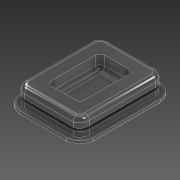
# Autodesk Inventor part: TAPAV2
Saved by Autodesk Inventor 2021 (Build 250183000, 183)
## iProperties
Created: 2022-08-14
Part Number: TAPAV2
Material: Plástico ABS
Document SubType Name: Modeling
Designer: PC
Density: 1.06 g/cm^3
Appearance: Gris oscuro
Author: PC
Autodesk Inventor part; units mm, degrees
ref_plane "YZ Plane" through (0, 0, 0) normal (1, 0, 0) x (0, 1, 0)
ref_plane "XZ Plane" through (0, 0, 0) normal (0, 1, 0) x (-1, 0, 0)
ref_plane "XY Plane" through (0, 0, 0) normal (0, 0, 1) x (1, 0, 0)
sketch "Boceto1" plane through (0, 0, 0) normal (0, 1, 0) x (-1, 0, 0)
  arc A0 (9.988, -9.8253) -> (15.988, -3.8253) centre (9.988, -3.8253) ccw
  line L0 (15.988, -3.8253) -> (15.988, 24.6747)
  arc A1 (15.988, 24.6747) -> (9.988, 30.6747) centre (9.988, 24.6747) ccw
  line L1 (9.988, 30.6747) -> (-9.862, 30.6747)
  arc A2 (-9.862, 30.6747) -> (-15.862, 24.6747) centre (-9.862, 24.6747) ccw
  line L2 (-15.862, 24.6747) -> (-15.862, -3.8253)
  arc A3 (-15.862, -3.8253) -> (-9.862, -9.8253) centre (-9.862, -3.8253) ccw
  line L3 (-9.862, -9.8253) -> (9.988, -9.8253)
  arc A4 (-13.862, -3.8253) -> (-9.862, -7.8253) centre (-9.862, -3.8253) ccw
  line L4 (-13.862, -3.8253) -> (-13.862, 24.6747)
  arc A5 (-10.9421, 28.6747) -> (-13.862, 24.6747) centre (-9.6623, 24.6747) ccw
  line L5 (-10.9421, 28.6747) -> (9.988, 28.6747)
  arc A6 (13.988, 24.6747) -> (9.988, 28.6747) centre (9.988, 24.6747) ccw
  line L6 (13.988, 24.6747) -> (13.988, -4.9054)
  arc A7 (9.988, -7.8253) -> (13.988, -4.9054) centre (9.988, -3.6255) ccw
  line L7 (9.988, -7.8253) -> (-9.862, -7.8253)
  line L8 (14.388, -4.9664) -> (14.388, 24.6747)
  arc A8 (14.388, 24.6747) -> (9.988, 29.0747) centre (9.988, 24.6747) ccw
  line L9 (9.988, 29.0747) -> (-11.0031, 29.0747)
  arc A9 (-11.0031, 29.0747) -> (-14.262, 24.6747) centre (-9.6623, 24.6747) ccw
  line L10 (-14.262, 24.6747) -> (-14.262, -3.8253)
  arc A10 (-14.262, -3.8253) -> (-9.862, -8.2253) centre (-9.862, -3.8253) ccw
  line L11 (-9.862, -8.2253) -> (9.988, -8.2253)
  arc A11 (9.988, -8.2253) -> (14.388, -4.9664) centre (9.988, -3.6255) ccw
  point P0 (0, 0)
  point P1 (0, 0)
  dimension "d0" = 27.85
  dimension "d1" = 40.5
  dimension "d2" = 6
  dimension "d3" = 2
  dimension "d4" = 2
  dimension "d5" = 2
  dimension "d6" = 2
  dimension "d7" = 2
  dimension "d8" = 0.4
  constraints: 24 end point, 24 point on circle, 12 centre point, 7 other
  measures "d0" distance between parallel lines of L4 L6
  measures "d1" distance between parallel lines of L3 L1
  measures "d2" radius of A0
  measures "d3" distance between parallel lines of L0 L6
  measures "d4" distance between parallel lines of L3 L7
  measures "d5" distance between parallel lines of L2 L4
  measures "d6" distance between parallel lines of L1 L5
  measures "d7" radial gap between concentric circles of A6 A1
  measures "d8" distance between parallel lines of L6 L8
extrude "Extrusión1" add sketch "Boceto1" along normal blind 4 contours L4 A5 L5 A6 L6 A7 L7 A4
extrude "Extrusión2" add sketch "Boceto1" along normal blind 2 contours L3 A3 L2 A2 L1 A1 L0 A0 | A11 L11 A10 L10 A9 L9 A8 L8
sketch "Boceto2" plane through (0, 4, 0) normal (0, 1, 0) x (1, 0, 0)
  line L0 (13.862, -24.6747) -> (13.862, 3.8253) projected
  arc A0 (13.862, 3.8253) -> (9.862, 7.8253) centre (9.862, 3.8253) ccw projected
  line L1 (9.862, 7.8253) -> (-9.988, 7.8253) projected
  arc A1 (-9.988, 7.8253) -> (-13.988, 4.9054) centre (-9.988, 3.6255) ccw projected
  line L2 (-13.988, 4.9054) -> (-13.988, -24.6747) projected
  arc A2 (-13.988, -24.6747) -> (-9.988, -28.6747) centre (-9.988, -24.6747) ccw projected
  line L3 (-9.988, -28.6747) -> (10.9421, -28.6747) projected
  arc A3 (10.9421, -28.6747) -> (13.862, -24.6747) centre (9.6623, -24.6747) ccw projected
  line L4 (-12.488, -24.6747) -> (-12.488, 4.6447)
  arc A4 (-9.988, 6.3253) -> (-12.488, 4.6447) centre (-9.988, 3.6255) ccw
  line L5 (-9.988, 6.3253) -> (9.862, 6.3253)
  arc A5 (12.362, 3.8253) -> (9.862, 6.3253) centre (9.862, 3.8253) ccw
  line L6 (12.362, 3.8253) -> (12.362, -24.6747)
  arc A6 (10.6815, -27.1747) -> (12.362, -24.6747) centre (9.6623, -24.6747) ccw
  line L7 (10.6815, -27.1747) -> (-9.988, -27.1747)
  arc A7 (-12.488, -24.6747) -> (-9.988, -27.1747) centre (-9.988, -24.6747) ccw
  point P0 (0, 0)
  dimension "d13" = 1.5
  constraints: 8 end point, 8 point on circle, 4 centre point, 7 other
  measures "d13" distance between parallel lines of L4 L2
extrude "Extrusión3" add sketch "Boceto2" along normal blind 1.3 contours L4 A4 L5 A5 L6 A6 L7 A7
sketch "Boceto3" plane through (0, 5.3, 0) normal (0, 1, 0) x (1, 0, 0)
  arc A0 (10.6815, -27.1747) -> (12.362, -24.6747) centre (9.6623, -24.6747) ccw projected
  line L0 (10.6815, -27.1747) -> (-9.988, -27.1747) projected
  arc A1 (-12.488, -24.6747) -> (-9.988, -27.1747) centre (-9.988, -24.6747) ccw projected
  line L1 (-12.488, -24.6747) -> (-12.488, 4.6447) projected
  arc A2 (-9.988, 6.3253) -> (-12.488, 4.6447) centre (-9.988, 3.6255) ccw projected
  line L2 (-9.988, 6.3253) -> (9.862, 6.3253) projected
  arc A3 (12.362, 3.8253) -> (9.862, 6.3253) centre (9.862, 3.8253) ccw projected
  line L3 (12.362, 3.8253) -> (12.362, -24.6747) projected
  line L4 (13.862, -24.6747) -> (13.862, 3.8253) projected
  arc A4 (13.862, 3.8253) -> (9.862, 7.8253) centre (9.862, 3.8253) ccw projected
  line L5 (9.862, 7.8253) -> (-9.988, 7.8253) projected
  arc A5 (-9.988, 7.8253) -> (-13.988, 4.9054) centre (-9.988, 3.6255) ccw projected
  line L6 (-13.988, 4.9054) -> (-13.988, -24.6747) projected
  arc A6 (-13.988, -24.6747) -> (-9.988, -28.6747) centre (-9.988, -24.6747) ccw projected
  line L7 (-9.988, -28.6747) -> (10.9421, -28.6747) projected
  arc A7 (10.9421, -28.6747) -> (13.862, -24.6747) centre (9.6623, -24.6747) ccw projected
  point P0 (0, 0)
extrude "Extrusión4" add sketch "Boceto3" along normal blind 4 contours L0 A1 L1 A2 L2 A3 L3 A0 | A7 L7 A6 L6 A5 L5 A4 L4
sketch "Boceto4" plane through (0, 9.3, 0) normal (0, 1, 0) x (1, 0, 0)
  arc A0 (13.862, 3.8253) -> (9.862, 7.8253) centre (9.862, 3.8253) ccw projected
  line L0 (9.862, 7.8253) -> (-9.988, 7.8253) projected
  arc A1 (-9.988, 7.8253) -> (-13.988, 4.9054) centre (-9.988, 3.6255) ccw projected
  line L1 (-13.988, 4.9054) -> (-13.988, -24.6747) projected
  arc A2 (-13.988, -24.6747) -> (-9.988, -28.6747) centre (-9.988, -24.6747) ccw projected
  line L2 (-9.988, -28.6747) -> (10.9421, -28.6747) projected
  arc A3 (10.9421, -28.6747) -> (13.862, -24.6747) centre (9.6623, -24.6747) ccw projected
  line L3 (13.862, -24.6747) -> (13.862, 3.8253) projected
  line L4 (-12.188, -24.6747) -> (-12.188, 4.5841)
  arc A4 (-9.988, 6.0253) -> (-12.188, 4.5841) centre (-9.988, 3.6255) ccw
  line L5 (-9.988, 6.0253) -> (9.862, 6.0253)
  arc A5 (12.062, 3.8253) -> (9.862, 6.0253) centre (9.862, 3.8253) ccw
  line L6 (12.062, 3.8253) -> (12.062, -24.6747)
  arc A6 (10.6209, -26.8747) -> (12.062, -24.6747) centre (9.6623, -24.6747) ccw
  line L7 (10.6209, -26.8747) -> (-9.988, -26.8747)
  arc A7 (-12.188, -24.6747) -> (-9.988, -26.8747) centre (-9.988, -24.6747) ccw
  line L8 (-7.2861, -0.8765) -> (-7.2861, -19.9729)
  line L9 (-5.2861, -21.9729) -> (5.1602, -21.9729)
  line L10 (7.1602, -19.9729) -> (7.1602, -0.8765)
  line L11 (5.1602, 1.1235) -> (-5.2861, 1.1235)
  arc A8 (-7.2861, -19.9729) -> (-5.2861, -21.9729) centre (-5.2861, -19.9729) ccw
  arc A9 (-5.2861, 1.1235) -> (-7.2861, -0.8765) centre (-5.2861, -0.8765) ccw
  arc A10 (7.1602, -0.8765) -> (5.1602, 1.1235) centre (5.1602, -0.8765) ccw
  arc A11 (5.1602, -21.9729) -> (7.1602, -19.9729) centre (5.1602, -19.9729) ccw
  point P0 (0, 0)
  dimension "d18" = 1.8
  dimension "d19" = 2
  constraints: 16 end point, 16 point on circle, 8 centre point, 8 tangent, 3 equal radius, 10 other
  measures "d18" distance between parallel lines of L4 L1
  measures "d19" radius of A8
extrude "Extrusión5" cut sketch "Boceto4" against normal blind 6 contours A9 L11 A10 L10 A11 L9 A8 L8
fillet "Empalme1" radius 2 8 edges at (-6.7003, 3.3, -0.5377) (-0.063, 3.3, -1.1235) (6.5744, 3.3, -0.5377) (7.1602, 3.3, 10.4247) (6.5744, 3.3, 21.3871) (-0.063, 3.3, 21.9729) (-6.7003, 3.3, 21.3871) (-7.2861, 3.3, 10.4247)
fillet "Empalme2" radius 2 8 edges at (-12.8164, 9.3, 27.5031) (-13.988, 9.3, 9.8847) (0.4771, 9.3, 28.6747) (-12.4641, 9.3, -7.0177) (12.6905, 9.3, -6.6537) (13.862, 9.3, 10.4247) (13.0544, 9.3, 27.1509) (-0.063, 9.3, -7.8253)
fillet "Empalme3" radius 1 8 edges at (-14.2306, 0, 28.9173) (-0.063, 0, 30.6747) (14.1047, 0, 28.9173) (15.862, 0, 10.4247) (14.1047, 0, -8.0679) (-0.063, 0, -9.8253) (-14.2306, 0, -8.0679) (-15.988, 0, 10.4247)
sketch "Boceto5" plane through (0, 0, 0) normal (0, -1, 0) x (1, 0, 0)
  line L0 (-2.8976, -4.217) -> (-2.8976, 9.8768) construction
  line L1 (-2.8976, 9.8768) -> (29.3615, 9.8768) construction
  line L2 (29.3615, 9.8768) -> (29.3615, -4.217) construction
  line L3 (29.3615, -4.217) -> (-2.8976, -4.217) construction
  line L4 (-2.8976, -3.5852) -> (-2.8976, -0.7989)
  spline S0 degree 2 poles (-2.8976, -0.7989) (-2.8976, -0.0973) (-2.7533, 0.7436) (-2.5941, 0.9923) knots 0 0 0 1 2 2 2
  spline S1 degree 2 poles (-2.5941, 0.9923) (-2.3304, 1.4053) (-1.4697, 1.8332) (-0.9124, 1.8332) knots 0 0 0 1 2 2 2
  spline S2 degree 2 poles (-0.9124, 1.8332) (-0.3651, 1.8332) (0.421, 1.4849) (0.6798, 1.1267) knots 0 0 0 1 2 2 2
  spline S3 degree 2 poles (0.6798, 1.1267) (0.8887, 0.8281) (1.0679, 0.052) (1.0679, -0.7491) knots 0 0 0 1 2 2 2
  line L5 (1.0679, -0.7491) -> (1.0679, -2.3015)
  line L6 (1.0679, -2.3015) -> (3.2024, -2.3015)
  line L7 (3.2024, -2.3015) -> (3.2024, -3.5852)
  line L8 (3.2024, -3.5852) -> (-2.8976, -3.5852)
  line L9 (-1.808, -0.8188) -> (-1.808, -2.3015)
  line L10 (-1.808, -2.3015) -> (-0.0118, -2.3015)
  line L11 (-0.0118, -2.3015) -> (-0.0118, -0.7392)
  spline S4 degree 2 poles (-0.0118, -0.7392) (-0.0118, -0.157) (-0.4547, 0.4052) (-0.9124, 0.4052) knots 0 0 0 1 2 2 2
  spline S5 degree 2 poles (-0.9124, 0.4052) (-1.4, 0.4052) (-1.808, -0.1471) (-1.808, -0.8188) knots 0 0 0 1 2 2 2
  line L12 (-2.8976, 3.9826) -> (0.7494, 3.9826)
  spline S6 degree 2 poles (0.7494, 3.9826) (1.6052, 3.9826) (2.2819, 4.5996) (2.2819, 5.3559) knots 0 0 0 1 2 2 2
  spline S7 degree 2 poles (2.2819, 5.3559) (2.2819, 6.1122) (1.6102, 6.7241) (0.7494, 6.7241) knots 0 0 0 1 2 2 2
  line L13 (0.7494, 6.7241) -> (-2.8976, 6.7241)
  line L14 (-2.8976, 6.7241) -> (-2.8976, 8.0078)
  line L15 (-2.8976, 8.0078) -> (0.7843, 8.0078)
  spline S8 degree 2 poles (0.7843, 8.0078) (1.4311, 8.0078) (2.2023, 7.8387) (2.4262, 7.6496) knots 0 0 0 1 2 2 2
  spline S9 degree 2 poles (2.4262, 7.6496) (2.8591, 7.2864) (3.267, 6.1768) (3.267, 5.3559) knots 0 0 0 1 2 2 2
  spline S10 degree 2 poles (3.267, 5.3559) (3.267, 4.5349) (2.8591, 3.4154) (2.4262, 3.0522) knots 0 0 0 1 2 2 2
  spline S11 degree 2 poles (2.4262, 3.0522) (2.2073, 2.8681) (1.4609, 2.7039) (0.7843, 2.7039) knots 0 0 0 1 2 2 2
  line L16 (0.7843, 2.7039) -> (-2.8976, 2.7039)
  line L17 (-2.8976, 2.7039) -> (-2.8976, 3.9826)
  spline S12 degree 2 poles (3.2024, 11.6698) (3.2024, 10.819) (2.9138, 9.9881) (2.5605, 9.6597) knots 0 0 0 1 2 2 2
  spline S13 degree 2 poles (2.5605, 9.6597) (2.2471, 9.3562) (1.451, 9.1074) (0.7295, 9.1074) knots 0 0 0 1 2 2 2
  line L18 (0.7295, 9.1074) -> (-2.8976, 9.1074)
  line L19 (-2.8976, 9.1074) -> (-2.8976, 10.3911)
  line L20 (-2.8976, 10.3911) -> (0.6847, 10.3911)
  spline S14 degree 2 poles (0.6847, 10.3911) (1.2221, 10.3911) (1.655, 10.4856) (1.7893, 10.6001) knots 0 0 0 1 2 2 2
  spline S15 degree 2 poles (1.7893, 10.6001) (2.0033, 10.7842) (2.1874, 11.3166) (2.1874, 11.7843) knots 0 0 0 1 2 2 2
  line L21 (2.1874, 11.7843) -> (2.1874, 13.2918)
  line L22 (2.1874, 13.2918) -> (3.2024, 13.2918)
  line L23 (3.2024, 13.2918) -> (3.2024, 11.6698)
  line L24 (-1.808, 19.1331) -> (-1.808, 15.9637)
  spline S16 degree 2 poles (-1.808, 15.9637) (-1.808, 15.4512) (-1.4249, 14.9736) (-1.0119, 14.9736) knots 0 0 0 1 2 2 2
  spline S17 degree 2 poles (-1.0119, 14.9736) (-0.6835, 14.9736) (-0.3502, 15.3816) (-0.3502, 15.7846) knots 0 0 0 1 2 2 2
  line L25 (-0.3502, 15.7846) -> (-0.3502, 17.4812)
  spline S18 degree 2 poles (-0.3502, 17.4812) (-0.3502, 18.5361) (0.4459, 19.4267) (1.3763, 19.4267) knots 0 0 0 1 2 2 2
  spline S19 degree 2 poles (1.3763, 19.4267) (2.3167, 19.4267) (3.2024, 18.3967) (3.2024, 17.2971) knots 0 0 0 1 2 2 2
  line L26 (3.2024, 17.2971) -> (3.2024, 13.879)
  line L27 (3.2024, 13.879) -> (2.1127, 13.879)
  line L28 (2.1127, 13.879) -> (2.1127, 17.0931)
  spline S20 degree 2 poles (2.1127, 17.0931) (2.1127, 17.6405) (1.7943, 18.0883) (1.4261, 18.0883) knots 0 0 0 1 2 2 2
  spline S21 degree 2 poles (1.4261, 18.0883) (1.043, 18.0883) (0.7196, 17.6753) (0.7196, 17.1777) knots 0 0 0 1 2 2 2
  line L29 (0.7196, 17.1777) -> (0.7196, 15.6652)
  spline S22 degree 2 poles (0.7196, 15.6652) (0.7196, 14.6104) (-0.1213, 13.6352) (-1.0318, 13.6352) knots 0 0 0 1 2 2 2
  spline S23 degree 2 poles (-1.0318, 13.6352) (-2.002, 13.6352) (-2.8976, 14.6601) (-2.8976, 15.7746) knots 0 0 0 1 2 2 2
  line L30 (-2.8976, 15.7746) -> (-2.8976, 19.1331)
  line L31 (-2.8976, 19.1331) -> (-1.808, 19.1331)
  spline S24 degree 2 poles (-1.8329, 22.9095) (-1.8329, 22.213) (-1.1363, 21.5015) (-0.4198, 21.4666) knots 0 0 0 1 2 2 2
  line L32 (-0.4198, 21.4666) -> (-0.4148, 25.0142)
  line L33 (-0.4148, 25.0142) -> (0.6449, 25.0142)
  line L34 (0.6449, 25.0142) -> (0.6449, 21.4567)
  spline S25 degree 2 poles (0.6449, 21.4567) (1.441, 21.4617) (2.1376, 22.1284) (2.1376, 22.9095) knots 0 0 0 1 2 2 2
  line L35 (2.1376, 22.9095) -> (2.1376, 25.0142)
  line L36 (2.1376, 25.0142) -> (3.2024, 25.0142)
  line L37 (3.2024, 25.0142) -> (3.2024, 22.8449)
  spline S26 degree 2 poles (3.2024, 22.8449) (3.2024, 22.1284) (2.9586, 21.3074) (2.665, 20.9442) knots 0 0 0 1 2 2 2
  spline S27 degree 2 poles (2.665, 20.9442) (2.2918, 20.4765) (1.0927, 20.0088) (0.2618, 20.0088) knots 0 0 0 1 2 2 2
  spline S28 degree 2 poles (0.2618, 20.0088) (-1.3602, 20.0088) (-2.8976, 21.4119) (-2.8976, 22.8847) knots 0 0 0 1 2 2 2
  line L38 (-2.8976, 22.8847) -> (-2.8976, 25.0142)
  line L39 (-2.8976, 25.0142) -> (-1.8329, 25.0142)
  line L40 (-1.8329, 25.0142) -> (-1.8329, 22.9095)
  point P0 (0, 0)
  constraints: 2 other
extrude "Extrusión6" cut sketch "Boceto5" against normal blind 0.3
fillet "Empalme4" radius 0.5 8 edges at (-11.7557, 5.3, 26.4425) (0.3468, 5.3, 27.1747) (-12.488, 5.3, 10.015) (-0.063, 5.3, -6.3253) (11.6298, 5.3, -5.5931) (12.362, 5.3, 10.4247) (11.9029, 5.3, 26.1809) (-11.4941, 5.3, -5.8661)
